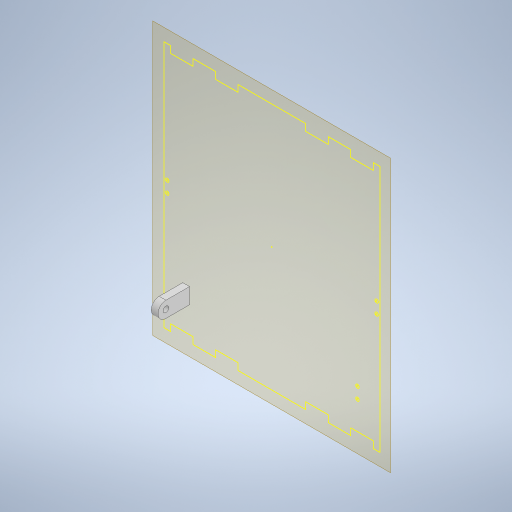
# Autodesk Inventor part: держатель вала
Saved by Autodesk Inventor 2024.2 (Build 282272000, 272)
## iProperties
Created: 2025-11-27
Part Number: держатель вала
Material: Типовые
Document SubType Name: Modeling
Designer: Zakhar
Density: 1 g/cm^3
Appearance: По умолчанию
Author: Zakhar
Autodesk Inventor part; units mm, degrees
ref_plane "YZ Plane" through (0, 0, 0) normal (1, 0, 0) x (0, 1, 0)
ref_plane "XZ Plane" through (0, 0, 0) normal (0, 1, 0) x (-1, 0, 0)
ref_plane "XY Plane" through (0, 0, 0) normal (0, 0, 1) x (1, 0, 0)
ref_plane "РабПлоскость1" through (0, 0, 0) normal (0, 0, 1) x (1, 0, 0)
sketch "Эскиз1" plane through (0, 0, 0) normal (0, 0, 1) x (1, 0, 0)
  circle A0 centre (-93, 5) radius 1.5 projected
  circle A1 centre (93, 5) radius 1.5 projected
  circle A2 centre (-93, -5) radius 1.5 projected
  circle A3 centre (93, -5) radius 1.5 projected
  line L0 (30, -110) -> (30, -104) projected
  line L1 (30, -104) -> (50, -104) projected
  line L2 (50, -104) -> (50, -110) projected
  line L3 (50, -110) -> (70, -110) projected
  line L4 (70, -110) -> (70, -104) projected
  line L5 (70, -104) -> (90, -104) projected
  line L6 (90, -104) -> (90, -110) projected
  line L7 (90, -110) -> (96, -110) projected
  line L8 (96, -110) -> (96, 110) projected
  line L9 (96, 110) -> (90, 110) projected
  line L10 (90, 110) -> (90, 104) projected
  line L11 (90, 104) -> (70, 104) projected
  line L12 (70, 104) -> (70, 110) projected
  line L13 (70, 110) -> (50, 110) projected
  line L14 (50, 110) -> (50, 104) projected
  line L15 (50, 104) -> (30, 104) projected
  line L16 (30, 104) -> (30, 110) projected
  line L17 (30, 110) -> (-30, 110) projected
  line L18 (-30, 110) -> (-30, 104) projected
  line L19 (-30, 104) -> (-50, 104) projected
  line L20 (-50, 104) -> (-50, 110) projected
  line L21 (-50, 110) -> (-70, 110) projected
  line L22 (-70, 110) -> (-70, 104) projected
  line L23 (-70, 104) -> (-90, 104) projected
  line L24 (-90, 104) -> (-90, 110) projected
  line L25 (-90, 110) -> (-96, 110) projected
  line L26 (-96, 110) -> (-96, -110) projected
  line L27 (-96, -110) -> (-90, -110) projected
  line L28 (-90, -110) -> (-90, -104) projected
  line L29 (-90, -104) -> (-70, -104) projected
  line L30 (-70, -104) -> (-70, -110) projected
  line L31 (-70, -110) -> (-50, -110) projected
  line L32 (-50, -110) -> (-50, -104) projected
  line L33 (-50, -104) -> (-30, -104) projected
  line L34 (-30, -104) -> (-30, -110) projected
  line L35 (-30, -110) -> (30, -110) projected
  circle A4 centre (76, -69) radius 1.5 projected
  circle A5 centre (76, -79) radius 1.5 projected
  circle A6 centre (-76, -69) radius 1.5 projected
  circle A7 centre (-76, -79) radius 1.5 projected
  point P0 (0, 0)
sketch "Эскиз2" plane through (0, 0, 0) normal (0, 0, 1) x (1, 0, 0)
  circle A0 centre (-76, -79) radius 1.5
  circle A1 centre (-76, -69) radius 1.5
  circle A2 centre (-76, -79) radius 1.5 projected
  circle A3 centre (-76, -69) radius 1.5 projected
  line L0 (-79, -81) -> (-73, -81)
  line L1 (-73, -81) -> (-73, -67)
  line L2 (-73, -67) -> (-79, -67)
  line L3 (-79, -67) -> (-79, -81)
  circle A4 centre (-76, -79) radius 1
  circle A5 centre (-76, -69) radius 1
  point P0 (0, 0)
  dimension "d0" = 3
  dimension "d1" = 3
  dimension "d2" = 14
  dimension "d3" = 2
  dimension "d4" = 2
  dimension "d5" = 2
  dimension "d6" = 6
  dimension "d7" = 3
  constraints: 8 end point, 4 centre point, 4 coincident, 2 parallel, 1 horizontal, 1 perpendicular
  measures "d0" diameter of A1
  measures "d1" diameter of A0
  measures "d2" distance of L2.end L0.start
  measures "d3" distance from line of L2 A1.centre
  measures "d4" diameter of A5
  measures "d5" diameter of A4
  measures "d6" distance between parallel lines of L1 L3
  measures "d7" distance from line of L1 A0.centre
extrude "Выдавливание1" add sketch "Эскиз2" along normal blind 16 contours A0 | A1 | L3 L2 L1 L0 | A4 | A5
extrude "Выдавливание6" cut sketch "Эскиз2" along normal blind 4 contours A0 | A1 | A4 | A5
thread "Резьба1" size "M3x0.5" class "6H" standard "ANSI Metric M Profile" full length
thread "Резьба2" size "M3x0.5" class "6H" standard "ANSI Metric M Profile" full length
sketch "Эскиз5" plane through (-73, -81, 0) normal (1, 0, 0) x (0, 0, -1)
  line L0 (-16, 0) -> (-16, 14) projected
  line L1 (-16, 0) -> (-21, 0)
  line L2 (-21, 0) -> (-21, 14)
  line L3 (-21, 14) -> (-16, 14)
  line L4 (-16, 14) -> (-16, 0)
  line L5 (0, 14) -> (-16, 14) projected
  circle A0 centre (-21, 7) radius 2.5
  circle A1 centre (-21, 7) radius 7
  point P0 (0, 81)
  point P1 (-21, 0)
  dimension "d30" = 5
  dimension "d31" = 5
  dimension "d32" = 7
  dimension "d33" = 14
  constraints: 8 end point, 2 centre point, 2 parallel, 1 coincident, 1 collinear, 1 horizontal, 1 midpoint, 1 perpendicular
  measures "d30" distance between parallel lines of L0 L2
  measures "d31" diameter of A0
  measures "d32" distance from line of L1 A0.centre
  measures "d33" diameter of A1
extrude "Выдавливание7" add sketch "Эскиз5" against normal blind 6 contours L1 A1 L0 | A1 L2 A0 L0 | A1 L2 A0 | A1 L3 L0
